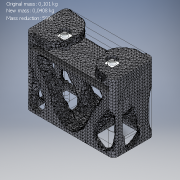
# Autodesk Inventor part: F550Spacer_down
Saved by Autodesk Inventor 2018.3 (Build 223284000, 284)
## iProperties
Created: 2019-01-03
Part Number: F550Spacer_down
Material: Genérico
Document SubType Name: Modeling
Designer: becar
Density: 1 g/cm^3
Appearance: Valor por defecto
Mass: 12.804 g
Surface Area: 68.848 cm^2
Volume: 12.804 cm^3
Author: becar
Autodesk Inventor part; units mm, degrees
ref_plane "YZ Plane" through (0, 0, 0) normal (1, 0, 0) x (0, 1, 0)
ref_plane "XZ Plane" through (0, 0, 0) normal (0, 1, 0) x (-1, 0, 0)
ref_plane "XY Plane" through (0, 0, 0) normal (0, 0, 1) x (1, 0, 0)
sketch "Boceto1" plane through (0, 0, 0) normal (0, 0, 1) x (1, 0, 0)
  line L0 (0, 0) -> (35.32, 0)
  line L1 (0, 0) -> (0, 15.33)
  line L2 (0, 15.33) -> (35.32, 15.33)
  line L3 (35.32, 15.33) -> (35.32, 0)
  dimension "d0" = 35.32
  dimension "d1" = 15.33
  constraints: 8 end point, 2 perpendicular, 1 horizontal, 1 vertical
  measures "d0" distance of L0.start L0.end
  measures "d1" distance of L0.start L1.end
extrude "Extrusión1" add sketch "Boceto1" along normal blind 20
sketch "Boceto2" plane through (0, 0, 0) normal (0, 0, -1) x (-1, 0, 0)
  line L0 (0, 15.33) -> (0, 0) projected
  line L1 (-35.32, 15.33) -> (0, 15.33) projected
  line L2 (-35.32, 0) -> (-35.32, 15.33) projected
  line L3 (-11.6, 2) -> (-11.6, 13.33)
  line L4 (-23.72, 2) -> (-23.72, 13.33)
  line L5 (-1, 2) -> (-1, 14.33)
  line L6 (-1, 14.33) -> (-11.6, 14.33)
  line L7 (-11.6, 14.33) -> (-11.6, 13.33)
  line L8 (-1, 2) -> (-1, 1)
  line L9 (-1, 1) -> (-11.468, 1)
  line L10 (-11.468, 1) -> (-11.6, 1)
  line L11 (-11.6, 1) -> (-11.6, 2)
  line L12 (-23.72, 2) -> (-23.72, 1)
  line L13 (-23.72, 1) -> (-34.32, 1)
  line L14 (-34.32, 1) -> (-34.32, 14.33)
  line L15 (-34.32, 14.33) -> (-23.72, 14.33)
  line L16 (-23.72, 14.33) -> (-23.72, 13.33)
  line L17 (0, 0) -> (-35.32, 0) projected
  line L18 (0, 0) -> (-35.32, 0)
  constraints: 30 end point, 5 perpendicular, 3 point on line, 2 parallel, 2 vertical, 1 horizontal
extrude "Extrusión2" add sketch "Boceto2" along normal blind 3
sketch "Boceto3" plane through (0, 0, 20) normal (0, 0, 1) x (1, 0, 0)
  line L0 (0, 0) -> (35.32, 0) projected
  line L1 (-1, 0) -> (-1, -1)
  line L2 (-1, -1) -> (35.32, -1)
  line L3 (35.32, -1) -> (36.32, -1)
  line L4 (36.32, -1) -> (36.32, 15.33)
  line L5 (36.32, 15.33) -> (36.32, 16.33)
  line L6 (36.32, 16.33) -> (-1, 16.33)
  line L7 (-1, 16.33) -> (-1, -1)
  line L8 (35.32, 15.33) -> (35.32, 0) projected
  line L9 (35.32, 0) -> (35.32, 15.33)
  line L10 (0, 15.33) -> (35.32, 15.33) projected
  line L11 (35.32, 15.33) -> (0, 15.33)
  line L12 (0, 15.33) -> (0, 0)
  dimension "d13" = 1
  dimension "d14" = 1
  dimension "d15" = 1
  dimension "d16" = 1
  constraints: 20 end point, 6 perpendicular, 3 point on line, 1 collinear
  measures "d13" distance of L0.start L1.start
  measures "d14" distance of L1.start L1.end
  measures "d15" distance of L2.end L3.end
  measures "d16" distance of L4.end L5.end
extrude "Extrusión3" add sketch "Boceto3" against normal blind 23
sketch "Boceto4" plane through (0, 0, 0) normal (0, 0, -1) x (-1, 0, 0)
  line L0 (-34.32, 14.33) -> (-23.72, 14.33) projected
  line L1 (-34.32, 14.33) -> (-33.32, 14.33)
  line L2 (-33.32, 14.33) -> (-23.72, 14.33)
  line L3 (-23.72, 14.33) -> (-24.72, 14.33)
  line L4 (-24.72, 14.33) -> (-24.72, 1)
  line L5 (-23.72, 1) -> (-34.32, 1) projected
  line L6 (-24.72, 14.33) -> (-24.72, 13.33)
  line L7 (-24.72, 1) -> (-24.72, 2)
  line L8 (-24.72, 2) -> (-24.72, 7)
  line L9 (-24.72, 7) -> (-27.72, 7)
  line L10 (-11.6, 1) -> (-11.6, 14.33) projected
  line L11 (-11.6, 1) -> (-10.6, 1)
  line L12 (-1, 1) -> (-11.6, 1) projected
  line L13 (-10.6, 1) -> (-10.6, 2)
  line L14 (-10.6, 2) -> (-10.6, 7)
  line L15 (-10.6, 7) -> (-7.6, 7)
  circle A0 centre (-27.72, 7) radius 1.25
  circle A1 centre (-7.6, 7) radius 1.25
  point P0 (0, 0)
  dimension "d19" = 1
  dimension "d20" = 1
  dimension "d21" = 1
  dimension "d22" = 1
  dimension "d23" = 5
  dimension "d24" = 3
  dimension "d25" = 1
  dimension "d26" = 3
  dimension "d27" = 2.5
  dimension "d28" = 2.5
  constraints: 24 end point, 8 point on line, 4 perpendicular, 2 centre point, 2 coincident, 1 collinear
  measures "d19" distance of L0.start L1.end
  measures "d20" distance of L0.end L3.end
  measures "d21" distance of L3.end L6.end
  measures "d22" distance of L4.end L7.end
  measures "d23" distance of L7.end L8.end
  measures "d24" distance of L8.end L9.end
  measures "d25" distance of L10.start L11.end
  measures "d26" distance of L14.end L15.end
  measures "d27" diameter of A0
  measures "d28" diameter of A1
extrude "Extrusión4" cut sketch "Boceto4" against normal blind 20
sketch "Boceto5" plane through (36.32, -1, 20) normal (1, 0, 0) x (0, 0, -1)
  line L0 (20, 9.25) -> (20, 6.75) projected
  line L1 (20, 6.75) -> (20, 9.25)
  line L2 (20, 9.25) -> (20, 11.25)
  line L3 (20, 2) -> (20, 15.33) projected
  line L4 (20, 6.75) -> (20, 4.75)
  line L5 (20, 4.75) -> (17, 4.75)
  line L6 (17, 4.75) -> (17, 11.25)
  line L7 (17, 11.25) -> (0, 11.25)
  line L8 (0, 0) -> (0, 17.33) projected
  line L9 (0, 11.25) -> (3, 11.25)
  line L10 (3, 11.25) -> (3, 4.75)
  line L11 (3, 4.75) -> (17, 4.75)
  point P0 (20, 1)
  dimension "d31" = 2
  dimension "d32" = 2
  dimension "d33" = 3
  dimension "d34" = 3
  constraints: 18 end point, 4 point on line, 3 perpendicular, 2 horizontal, 1 vertical
  measures "d31" distance of L0.start L2.end
  measures "d32" distance of L0.end L4.end
  measures "d33" distance of L2.end L6.end
  measures "d34" distance of L7.end L9.end
extrude "Extrusión5" cut sketch "Boceto5" against normal blind 12.6
sketch "Boceto6" plane through (-1, -1, 20) normal (-1, 0, 0) x (0, 0, 1)
  line L0 (-20, 6.75) -> (-20, 9.25) projected
  line L1 (-20, 9.25) -> (-20, 6.75)
  line L2 (-20, 6.75) -> (0, 6.75) projected
  line L3 (-20, 6.75) -> (-20, 4.75)
  line L4 (-20, 4.75) -> (-17, 4.75)
  line L5 (-17, 4.75) -> (-17, 9.25)
  line L6 (-17, 11.25) -> (-17, 4.75) projected
  line L7 (-17, 9.25) -> (-17, 12.25)
  line L8 (-2.5, 11.25) -> (-2.5, 4.75)
  line L9 (-17, 12.25) -> (-2.5, 12.25)
  line L10 (-2.5, 12.25) -> (-2.5, 11.25)
  line L11 (-17, 4.75) -> (-17, 3.75)
  line L12 (-17, 3.75) -> (-2.5, 3.75)
  line L13 (-2.5, 3.75) -> (-2.5, 4.75)
  point P0 (-20, 1)
  point P1 (-3, 11.25)
  dimension "d37" = 2
  dimension "d38" = 3
  dimension "d39" = 3
  dimension "d43" = 0.5
  dimension "d58" = 1
  constraints: 22 end point, 4 vertical, 3 horizontal, 3 point on line, 2 perpendicular
  measures "d37" distance of L2.start L3.end
  measures "d38" distance of L3.end L4.end
  measures "d39" distance of L5.end L7.end
  measures "d43" distance of point (-3, 11.25) L8.start
  measures "d58" distance of L4.end L11.end
extrude "Extrusión6" cut sketch "Boceto6" against normal blind 12.6 contours L5 L6 L7 L9 L10 L8 L2 | L2 L8 L13 L12 L11 L5
sketch "Boceto7" plane through (-1, -1, 20) normal (0, -1, 0) x (1, 0, 0)
  line L0 (0, 0) -> (37.32, 0) projected
  line L1 (37.32, 0) -> (37.32, 2.5003)
  line L2 (37.32, 2.5003) -> (37.32, 5.5003)
  line L3 (37.32, 5.5003) -> (0, 5.5003)
  line L4 (0, 5.5003) -> (0, 0)
  line L5 (37.32, 2.5003) -> (0, 2.5003)
  line L6 (37.32, 0) -> (35.32, 0)
  line L7 (35.32, 0) -> (35.32, 2.5003)
  line L8 (0, 0) -> (2, 0)
  line L9 (2, 0) -> (2, 2.5003)
  point P0 (1, -20)
  dimension "d42" = 3
  dimension "d44" = 2
  dimension "d45" = 2
  constraints: 18 end point, 6 point on line, 5 perpendicular, 1 vertical
  measures "d42" distance of L1.end L2.end
  measures "d44" distance of L0.end L6.end
  measures "d45" distance of L0.start L8.end
extrude "Extrusión7" add sketch "Boceto7" against normal up to surface (17.33 mm away) contours L4 L5 L9 L0 | L4 L3 L2 L5 | L7 L5 L1 L0
sketch "Boceto8" plane through (0, 0, 20) normal (0, 0, 1) x (1, 0, 0)
  circle A0 centre (27.72, 7) radius 1.25 projected
  circle A1 centre (27.72, 7) radius 1.25
  circle A2 centre (7.6, 7) radius 1.25 projected
  circle A3 centre (7.6, 7) radius 1.25
  point P0 (0, 0)
  constraints: 2 centre point, 2 coincident
extrude "Extrusión8" cut sketch "Boceto8" along normal up to surface (5.5003 mm away)
sketch "Boceto9" plane through (-1, -1, 25.5003) normal (0, 0, 1) x (1, 0, 0)
  circle A0 centre (28.72, 8) radius 1.25 projected
  circle A1 centre (28.72, 8) radius 1.5
  circle A2 centre (8.6, 8) radius 1.25 projected
  circle A3 centre (8.6, 8) radius 1.5
  point P0 (1, 1)
  dimension "d50" = 3
  dimension "d51" = 3
  constraints: 2 centre point, 2 coincident
  measures "d50" diameter of A1
  measures "d51" diameter of A3
extrude "Extrusión9" cut sketch "Boceto9" against normal up to surface (25.5003 mm away)
sketch "Boceto10" plane through (-1, -1, 25.5003) normal (0, 0, 1) x (1, 0, 0)
  circle A0 centre (8.6, 8) radius 1.5 projected
  circle A1 centre (8.6, 8) radius 2
  circle A2 centre (28.72, 8) radius 1.5 projected
  circle A3 centre (28.72, 8) radius 2
  point P0 (1, 1)
  dimension "d54" = 4
  dimension "d55" = 4
  constraints: 2 centre point, 2 coincident
  measures "d54" diameter of A1
  measures "d55" diameter of A3
extrude "Extrusión10" cut sketch "Boceto10" against normal up to surface (8.5003 mm away)
sketch "Boceto11" plane through (36.32, -1, -3) normal (1, 0, 0) x (0, 0, -1)
  line L0 (-6, 11.25) -> (-6, 12.25)
  line L1 (-6, 12.25) -> (-20, 12.25)
  line L2 (-20, 11.25) -> (-6, 11.25) projected
  line L3 (-20, 12.25) -> (-20, 11.25)
  line L4 (-6, 11.25) -> (-6, 4.75) projected
  line L5 (-6, 3.75) -> (-6, 12.25) projected
  line L6 (-6, 4.75) -> (-6, 3.75)
  line L7 (-6, 3.75) -> (-20, 3.75)
  line L8 (-6, 4.75) -> (-20, 4.75) projected
  line L9 (-20, 3.75) -> (-20, 4.75)
  point P0 (-3, 1)
  dimension "d59" = 1
  dimension "d60" = 1
  constraints: 12 end point, 4 perpendicular, 2 vertical
  measures "d59" distance of L0.start L0.end
  measures "d60" distance of L4.end L5.start
extrude "Extrusión11" cut sketch "Boceto11" against normal blind 12.6
fillet "Empalme1" radius 2 4 edges at (36.32, -1, 11.2502) (36.32, 16.33, 11.2502) (-1, -1, 11.2502) (-1, 16.33, 11.2502)
